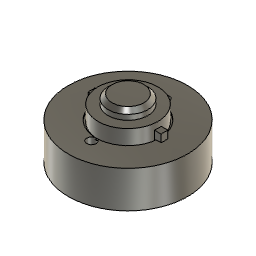
sphere_PS1 v10 (Autodesk Fusion 360 design; units mm, degrees)
Autodesk Fusion 360 part; units mm, degrees
sketch "Skizze1" plane through (0, 0, 0) normal (0, 0, 1) x (1, 0, 0)
  circle A0 centre (0, 0) radius 15
  circle A1 centre (0, 0) radius 1.7
  circle A2 centre (0, 0) radius 7.55
  line L0 (0, 17.9163) -> (0, -17.3071) construction
  circle A3 centre (0, 0) radius 9.2 construction
  circle A4 centre (0, 9.2) radius 1.2
  circle A5 centre (0, -9.2) radius 1.2
  circle A6 centre (0, 0) radius 5
  circle A7 centre (0, 0) radius 14.1421 construction
  line L1 (9.2, -0.85) -> (7.502, -0.85)
  line L2 (9.2, 0.85) -> (7.502, 0.85)
  line L3 (19.7442, 0) -> (-23.5704, 0) construction
  line L4 (-4.9272, -0.85) -> (-9.2, -0.85)
  line L5 (-4.9272, 0.85) -> (-9.2, 0.85)
  line L6 (-9.2, -0.85) -> (-9.2, 0.85)
  line L7 (9.2, -0.85) -> (9.2, 0.85)
  circle A8 centre (0, 0) radius 8
  point P0 (0, 9.2)
  point P1 (0, -9.2)
  dimension "d1" = 30
  dimension "d2" = 3.4
  dimension "d3" = 15.1
  dimension "d19" = 18.4
  dimension "d20" = 2.4
  dimension "d21" = 2.4
  dimension "d25" = 10
  dimension "d43" = 28.2843
  dimension "d58" = 0.85
  dimension "d59" = 0.85
  dimension "d60" = 0.85
  dimension "d61" = 0.85
  dimension "d62" = 9.2
  dimension "d63" = 9.2
  dimension "d66" = 16
  constraint coincident A0.centre A1.centre
  constraint concentric A0 A1
  constraint concentric A0 A2
  constraint vertical L0
  constraint coincident A3 P0
  constraint coincident L0 P0
  constraint coincident A3 P1
  constraint coincident L0 P1
  constraint coincident P0 A4.centre
  constraint coincident P1 A5.centre
  constraint concentric A1 A6
  constraint concentric A6 A7
  constraint horizontal L1
  constraint horizontal L2
  constraint horizontal L3
  constraint coincident A0.centre L3
  constraint coincident A2 L1.end
  constraint coincident A2 L2.end
  constraint parallel L3 L4
  constraint horizontal L5
  constraint coincident A6 L4.start
  constraint coincident A6 L5.start
  constraint vertical L6
  constraint perpendicular L3 L7
  constraint coincident L5 L6.end
  constraint coincident L4 L6.start
  constraint coincident L4.end L6
  constraint coincident L5.end L6
  constraint coincident L1.start L7
  constraint coincident L2.start L7
  constraint coincident L2 L7.end
  constraint coincident L1 L7.start
  measures "d1" diameter of A0
  measures "d2" diameter of A1
  measures "d3" diameter of A2
  measures "d19" diameter of A3
  measures "d20" diameter of A5
  measures "d21" diameter of A4
  measures "d25" diameter of A6
  measures "d43" diameter of A7
  measures "d58" distance of L1 L3
  measures "d59" distance of L2 L3
  measures "d60" distance of L3 L5
  measures "d61" distance of L3 L4
  measures "d62" distance of A0.centre L7
  measures "d63" distance of A0.centre L6
  measures "d66" diameter of A8
extrude "Extrusion1" add sketch "Skizze1" along normal blind 15 contours A1 | A6 makes body 1
extrude "Extrusion2" cut sketch "Skizze1" along normal blind 14 contours A1 bodies 1
extrude "Extrusion5" add sketch "Skizze1" along normal blind 12.7 contours A2 A6 L4 L5 | A2 A6 L4 L5 bodies 1
extrude "Extrusion9" add sketch "Skizze1" along normal blind 11.2 contours A2 L1 L2 A8 | A2 L4 L5 A8 | L1 L2 L7 A8 | L4 L5 L6 A8 bodies 1
extrude "Extrusion3" add sketch "Skizze1" along normal blind 9.3 separate body contours A0 | A2 L1 L2 A8 | A2 L4 L5 A8 | L1 L2 L7 A8 | L4 L5 L6 A8 makes body 2
extrude "Extrusion10" add sketch "Skizze1" along normal blind 8.8 contours A2 L2 L5 A8 | A2 L1 L4 A8 bodies 1 2
ref_plane "Arbeitsebene1" through (0, 0, 7.5) normal (0, 0, -1) x (-1, 0, 0)
sketch "Skizze2" plane through (0, 0, 7.5) normal (0, 0, -1) x (-1, 0, 0)
  line L0 (0, 19.4975) -> (0, -17.4097) construction
  line L1 (-20.2047, 0) -> (24.515, 0) construction
  circle A0 centre (0, 0) radius 9.2 construction
  line L2 (-1.3568, 11.55) -> (-2.7135, 9.2)
  line L3 (-2.7135, 9.2) -> (-1.3568, 6.85)
  line L4 (-1.3568, 6.85) -> (1.3568, 6.85)
  line L5 (1.3568, 6.85) -> (2.7135, 9.2)
  line L6 (2.7135, 9.2) -> (1.3568, 11.55)
  line L7 (1.3568, 11.55) -> (-1.3568, 11.55)
  line L8 (1.3568, -11.55) -> (2.7135, -9.2)
  line L9 (2.7135, -9.2) -> (1.3568, -6.85)
  line L10 (1.3568, -6.85) -> (-1.3568, -6.85)
  line L11 (-1.3568, -6.85) -> (-2.7135, -9.2)
  line L12 (-2.7135, -9.2) -> (-1.3568, -11.55)
  line L13 (-1.3568, -11.55) -> (1.3568, -11.55)
  point P0 (0, 9.2)
  point P1 (0, -9.2)
  point P2 (0, 9.2)
  point P3 (0, -9.2)
  dimension "d9" = 18.4
  dimension "d10" = 4.7
  dimension "d11" = 4.7
  constraint vertical L0
  constraint coincident L0 A0.centre
  constraint horizontal L1
  constraint coincident L1 A0.centre
  constraint coincident A0.centre origin
  constraint coincident A0 P2
  constraint coincident L0 P2
  constraint coincident A0 P3
  constraint coincident L0 P3
  constraint coincident P2 P0
  constraint coincident P3 P1
  measures "d9" diameter of A0
  measures "d10" distance of L10 L13
  measures "d11" distance of L4 L7
extrude "Extrusion4" cut sketch "Skizze2" along normal blind 2.1 bodies 1
chamfer "Fase2" distance 1 angle 45 1 edges at (-4.6616, -1.8081, 15) on bodies 1
